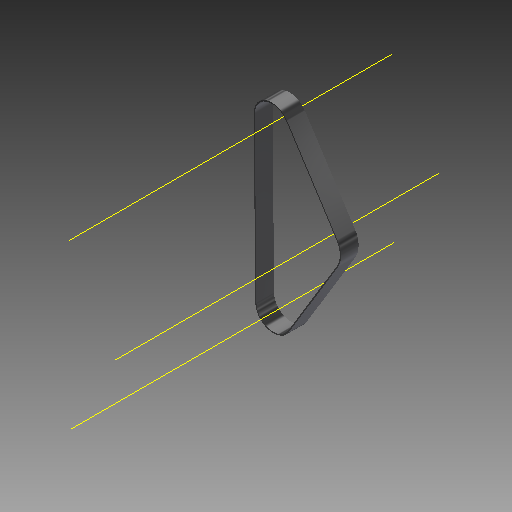
# Autodesk Inventor part: Synchronous Belt
Saved by Autodesk Inventor 2019.4 (Build 234330000, 330)
## iProperties
Created: 2020-01-06
Part Number: Synchronous Belt
Material: Rubber
Document SubType Name: Modeling
Designer: admin
Density: 1 g/cm^3
Appearance: Rubber - Black - Version 1.1
CustomPartVersion: 1
Author: admin
Autodesk Inventor part; units mm, degrees
sketch "Sketch Path" plane through (0, 0, 0) normal (0, 0, 1) x (1, 0, 0)
  arc A0 (-40.3012, -17.2737) -> (-10.7789, -25.3854) centre (-24.3863, -17.1306) ccw
  arc A1 (-12.3333, 138.5509) -> (-41.6232, 129.7817) centre (-25.7084, 129.9247) ccw
  arc A2 (33.259, 47.2082) -> (32.9686, 68.3094) centre (16.2497, 57.5267) ccw
  line L0 (33.259, 47.2082) -> (-10.7789, -25.3854)
  line L1 (-40.3012, -17.2737) -> (-41.6232, 129.7817)
  line L2 (-12.3333, 138.5509) -> (32.9686, 68.3094)
  constraints: 6 end point, 6 point on circle, 3 centre point
ref_plane "Cross Section Plane" through (-10.7789, -25.3854, 0) normal (0.5187, 0.855, 0) x (0, 0, 1)
ref_plane "Work Plane2" through (-24.3863, -17.1306, 0) normal (-1, 0, 0) x (0, 0, 1)
ref_plane "Work Plane3" through (-25.7084, 129.9247, 0) normal (-0.1836, -0.983, 0) x (0, 0, 1)
ref_plane "Work Plane4" through (16.2497, 57.5267, 0) normal (-0.3878, 0.9217, 0) x (0, 0, 1)
sketch "Cross Section" plane through (-10.7789, -25.3854, 0) normal (0.5187, 0.855, 0) x (0, 0, 1)
  line L0 (-8, 0.5) -> (8, 0.5)
  line L1 (8, 0.5) -> (8, -0.5)
  line L2 (8, -0.5) -> (-8, -0.5)
  line L3 (-8, -0.5) -> (-8, 0.5)
  line L4 (-8, 0) -> (8, 0) construction
  point P0 (0, 0)
  point P1 (0, 0)
  dimension "d0" = 16
  dimension "d4" = 0.5
  dimension "d5" = 0.5
  constraints: 10 end point, 3 midpoint, 2 parallel, 1 coincident, 1 horizontal, 1 perpendicular, 1 other
  measures "d0" distance between parallel lines of L1 L3
  measures "d4" distance between parallel lines of L2 L4
  measures "d5" distance between parallel lines of L4 L0
sweep "Belt" add profiles "Cross Section" path "Sketch Path"
equation "\"d0\" = da_B"
equation "\"d4\" = da_a"
equation "\"d5\" = da_a2"
equation "\"da_B\" = 16"
equation "\"da_pb\" = 5"
equation "\"da_a\" = 0.5"
equation "\"da_S\" = 2.65"
equation "\"da_Beta\" = 20deg"
equation "\"da_Ht\" = 1.2"
equation "\"da_H\" = 2.2"
equation "\"da_a2\" = 0.5"
body "Solid1"
